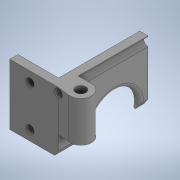
# Autodesk Inventor part: tool dock
Saved by Autodesk Inventor 2022 (Build 260153000, 153)
## iProperties
Created: 2021-11-28
Part Number: tool dock
Material: Polycarbonate, Clear
Document SubType Name: Modeling
Designer: alexr
Density: 1.2 g/cm^3
Appearance: Polycarbonate - Clear
Mass: 12.1555 g
Surface Area: 56.4567 cm^2
Volume: 10.1295 cm^3
Author: alexr
Autodesk Inventor part; units mm, degrees
ref_plane "YZ Plane" through (0, 0, 0) normal (1, 0, 0) x (0, 1, 0)
ref_plane "XZ Plane" through (0, 0, 0) normal (0, 1, 0) x (-1, 0, 0)
sketch "Sketch1" plane through (0, 0, 0) normal (0, 0, 1) x (1, 0, 0)
  line L0 (10, 0) -> (10, -500) projected
  line L1 (-10, 0) -> (-10, -500) projected
  line L2 (13.8571, -62.3) -> (-6.0929, -62.3) projected
  line L3 (10, -62.3) -> (-10, -62.3)
  line L4 (-10, -62.3) -> (-10, -92.3)
  line L5 (-10, -92.3) -> (10, -92.3)
  line L6 (10, -92.3) -> (10, -62.3)
  circle A0 centre (0, -87.3) radius 2
  circle A1 centre (0, -67.3) radius 2
  point P0 (0, 0)
  dimension "d0" = 30
  dimension "d1" = 4
  dimension "d2" = 4
  dimension "d3" = 5
  dimension "d4" = 5
  constraints: 8 end point, 3 point on line, 2 centre point, 2 parallel, 1 horizontal, 1 perpendicular
  measures "d0" distance of L4.end L3.end
  measures "d1" diameter of A0
  measures "d2" diameter of A1
  measures "d3" distance from line of L2 A1.centre
  measures "d4" distance from line of L5 A0.centre
extrude "Extrusion1" add sketch "Sketch1" along normal blind 4
ref_plane "Work Plane1" through (-10, -77.3, 0) normal (0, 1, 0) x (1, 0, 0)
sketch "Sketch3" plane through (10, -92.3, 0) normal (1, 0, 0) x (0, 0, -1)
  line L0 (0, 0) -> (0, 30) projected
  line L1 (0, 30) -> (-4, 30) projected
  line L2 (-4, 0) -> (-4, 30) projected
  line L3 (0, 0) -> (-4, 0) projected
  line L4 (0, 0) -> (0, 30) projected
  line L5 (0, 0) -> (20, 0)
  line L6 (20, 0) -> (20, 30)
  line L7 (20, 30) -> (0, 30)
  line L8 (0, 30) -> (0, 0)
  circle A0 centre (10, 25) radius 2
  circle A1 centre (10, 5) radius 2
  point P0 (0, 92.3)
  dimension "d12" = 20
  dimension "d13" = 4
  dimension "d14" = 4
  dimension "d15" = 5
  dimension "d16" = 5
  constraints: 8 end point, 2 centre point, 2 parallel, 1 horizontal, 1 perpendicular
  measures "d12" distance of L7.end L6.end
  measures "d13" diameter of A0
  measures "d14" diameter of A1
  measures "d15" distance from line of L5 A1.centre
  measures "d16" distance from line of L7 A0.centre
extrude "Extrusion3" add sketch "Sketch3" along normal blind 4 contours L3 L2 L1 L0 | L0 L7 L6 L5 | A0 | A1
sketch "Sketch2" plane through (-10, -77.3, 0) normal (0, 1, 0) x (1, 0, 0)
  line L0 (20, -4) -> (0, -4) projected
  line L1 (20, 0) -> (0, 0) projected
  line L2 (0, 0) -> (0, -4) projected
  line L3 (0, -4) -> (24, -4) projected
  line L4 (24, 20) -> (24, -4) projected
  line L5 (20, 20) -> (24, 20) projected
  line L6 (20, 20) -> (20, 0) projected
  line L7 (24, -4) -> (24, 20) projected
  circle A0 centre (30.5, 0.4456) radius 2.5
  circle A1 centre (30.5, 0.4456) radius 5.25
  line L8 (24, 20) -> (34.8957, 3.3163)
  line L9 (24, -4) -> (29.82, -4.7602)
  line L10 (30.5, 5.6956) -> (24, 5.6956)
  point P0 (10, 0)
  point P1 (24, 0.4456)
  dimension "d26" = 5
  dimension "d27" = 2.75
  dimension "d29" = 4.4456
  dimension "d30" = 6.5
  dimension "d50" = 10.5
  constraints: 6 end point, 3 point on circle, 3 tangent, 2 centre point, 1 perpendicular, 1 point on line
  measures "d26" diameter of A0
  measures "d27" radial gap between concentric circles of A0 A1
  measures "d29" distance from line of L3 A0.centre
  measures "d30" distance from line of L4 A0.centre
  measures "d50" diameter of A1
extrude "Extrusion2" add sketch "Sketch2" along normal mid plane 10 contours L4 L10 A1 L9 | A1
sketch "Sketch4" plane through (-10, -72.3, 0) normal (0, 1, 0) x (1, 0, 0)
  line L0 (23.958, -4) -> (24, -4) projected
  line L1 (24, -4) -> (24, -8.9113)
  arc A0 (29.82, -4.7602) -> (30.5, 5.6956) centre (30.5, 0.4456) ccw projected
  circle A1 centre (30.5, 0.4456) radius 2.5 projected
  line L2 (30.5, 5.6956) -> (24, 5.6956) projected
  line L3 (24, -4) -> (24, 5.6956) projected
  line L4 (24, -4) -> (29.82, -4.7602) projected
  point P0 (10, 0)
  point P1 (0, -4)
  point P2 (24, -4.0444)
  constraints: 2 end point, 1 vertical
extrude "Extrusion4" add sketch "Sketch4" along normal blind 10
fillet "Fillet1" [suppressed]
sketch "Sketch5" plane through (-10, -62.3, 4) normal (0, 1, 0) x (1, 0, 0)
  circle A0 centre (30.5, 4.4456) radius 2.5 projected
  line L0 (20, 24) -> (22, 44)
  line L1 (22, 44) -> (24, 44)
  line L2 (24, 44) -> (21.9516, 23.5162)
  line L3 (20, 24) -> (24, 24) projected
  point P0 (10, 4)
  point P1 (22, 24)
  dimension "d38" = 2
  dimension "d39" = 6.5
  dimension "d40" = 20
  constraints: 6 end point, 1 horizontal, 1 parallel
  measures "d38" distance of L0.end L1.end
  measures "d39" horizontal distance of L1.end A0.centre
  measures "d40" distance between parallel lines of L3 L1
extrude "Extrusion5" [suppressed]
fillet "Fillet2" [suppressed]
sketch "Sketch6" plane through (0, 0, 4) normal (0, 0, 1) x (1, 0, 0)
  circle A0 centre (14, -64.8) radius 2.1
  line L0 (25.7065, -62.3) -> (14, -62.3) projected
  line L1 (10, -92.3) -> (10, -62.3) projected
  line L2 (18, -62.3) -> (18, -82.3) projected
  line L3 (23, -62.3) -> (23, -96.3)
  line L4 (19.3, -67.6) -> (49.3, -67.6) projected
  line L5 (19.45, -67.3) -> (49.45, -67.3) projected
  point P0 (0, 0)
  dimension "d42" = 4.2
  dimension "d43" = 2.5
  dimension "d44" = 4
  constraints: 2 end point, 1 centre point, 1 vertical, 2 other
  measures "d42" diameter of A0
  measures "d43" distance from line of L0 A0.centre
  measures "d44" distance from line of L1 A0.centre
extrude "Extrusion6" cut sketch "Sketch6" along normal mid plane 100
chamfer "Chamfer1" distance 3 distance2 2 1 edges at (14, -92.3, -8) measured on face at (14, -80.5, -15.2319)
sketch "Sketch7" plane through (10, -92.3, -20) normal (0, 0, -1) x (-1, 0, 0)
  line L0 (-2, 0) -> (-4, 3) projected
  line L1 (0, 0) -> (-2, 0) projected
  line L2 (0, 0) -> (0, 30) projected
  line L3 (0, 30) -> (-4, 30) projected
  line L4 (-4, 29.6) -> (-4, 30) projected
  arc A0 (-4, 25.4) -> (-4, 29.6) centre (-4, 27.5) ccw projected
  line L5 (-4, 3) -> (-4, 25.4) projected
  point P0 (10, 92.3)
extrude "Extrusion7" add sketch "Sketch7" along normal blind 20
sketch "Sketch8" plane through (14, -92.3, 0) normal (1, 0, 0) x (0, 0, -1)
  line L0 (2.9456, 30) -> (2.9456, 10) projected
  line L1 (-2.0544, 30) -> (-2.0544, 10) projected
  circle A0 centre (23.9956, 2.25) radius 12
  line L2 (5.6956, 10) -> (-4, 10) projected
  point P0 (0, 92.3)
  point P1 (0.4456, 12.1254)
  dimension "d53" = 5
  dimension "d54" = 2.5
  dimension "d55" = 24
  dimension "d56" = 7.75
  dimension "d57" = 23.55
  constraints: 1 centre point
  measures "d53" distance between parallel lines of L1 L0
  measures "d54" distance from line of point (0.446, 12.125) L0
  measures "d55" diameter of A0
  measures "d56" distance from line of L2 A0.centre
  measures "d57" horizontal distance of A0.centre point (0.446, 12.125)
extrude "Extrusion8" cut sketch "Sketch8" against normal blind 10
fillet "Fillet3" radius 2 2 edges at (10, -78.05, -23.9956) (14, -78.05, -23.9956)
equation "\"d16\" = d15"
equation "\"d54\" = 0.5 * d53"
equation "\"d7\" = -0.5 * d0"
body "Solid1"
